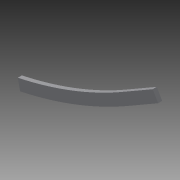
# Autodesk Inventor part: nd-l
Saved by Autodesk Inventor 2015 (Build 190159000, 159)
## iProperties
Created: 2014-07-02
Part Number: nd-l
Material: Generic
Document SubType Name: Modeling
Designer: peter
Density: 1 g/cm^3
Appearance: Default
Author: peter
Autodesk Inventor part; units mm, degrees
ref_plane "YZ Plane" through (0, 0, 0) normal (1, 0, 0) x (0, 1, 0)
ref_plane "XZ Plane" through (0, 0, 0) normal (0, 1, 0) x (-1, 0, 0)
ref_plane "XY Plane" through (0, 0, 0) normal (0, 0, 1) x (1, 0, 0)
sketch "Sketch1" plane through (0, 0, 0) normal (0, 0, 1) x (1, 0, 0)
  line L0 (655.3348, 274.2577) -> (523.3525, 198.0577)
  arc A0 (10.5239, 0.0422) -> (523.3525, 198.0577) centre (-347.2791, 1689.775) ccw
  line L1 (10.5239, 0.0422) -> (0.0003, 49.7403)
  arc A1 (0.0003, 49.7403) -> (497.8482, 241.9916) centre (-347.2791, 1689.775) ccw
  line L2 (497.8482, 241.9916) -> (629.9348, 318.2518)
  line L3 (629.9348, 318.2518) -> (655.3348, 274.2577)
  point P0 (0, 0)
  constraints: 8 end point, 4 point on circle, 2 centre point
extrude "Extrusion1" add sketch "Sketch1" along normal blind 19.05
body "Solid1"
